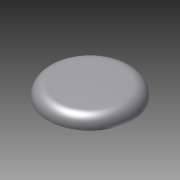
# Autodesk Inventor part: frisbee
Saved by Autodesk Inventor 2011 SP1 (Build 150282100, 282)
## iProperties
Created: 2013-01-26
Part Number: frisbee
Document SubType Name: Modeling
Designer: wes
Density: 1 g/cm^3
Author: wes
Autodesk Inventor part; units mm, degrees
ref_plane "YZ Plane" through (0, 0, 0) normal (1, 0, 0) x (0, 1, 0)
ref_plane "XZ Plane" through (0, 0, 0) normal (0, 1, 0) x (-1, 0, 0)
ref_plane "XY Plane" through (0, 0, 0) normal (0, 0, 1) x (1, 0, 0)
sketch "Sketch1" plane through (0, 0, 0) normal (0, 0, 1) x (1, 0, 0)
  line L0 (-25.5689, -10.4652) -> (78.4842, -10.4652)
  arc A0 (114.1311, -47.2952) -> (78.4842, -10.4652) centre (78.4842, -46.1311) ccw
  arc A1 (110.9543, -47.2952) -> (78.4842, -13.6402) centre (78.4842, -46.1311) ccw
  line L1 (78.4842, -13.6402) -> (-25.5689, -13.6402)
  line L2 (-25.5689, -13.6402) -> (-25.5689, -10.4652)
  line L3 (110.9543, -47.2952) -> (114.1311, -47.2952)
  point P0 (0, 0)
  dimension "d0" = 139.7
  dimension "d1" = 36.83
  dimension "d2" = 3.175
  constraints: 8 end point, 4 point on circle, 2 centre point, 2 perpendicular, 1 horizontal, 1 tangent, 1 other
  measures "d0" horizontal distance of L3.end L0.start
  measures "d1" distance from line of L3.end L0
  measures "d2" distance between parallel lines of L0 L1
revolve "Revolution1" add sketch "Sketch1" angle 360 about axis through (-25.5689, -13.6402, 0) along (0, 1, 0)
body "Solid1"
